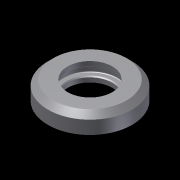
# Autodesk Inventor part: 機械油封墊片-KMB601PT-t10.4
Saved by Autodesk Inventor 2012 SP2 (Build 160219200, 219)
## iProperties
Created: 2015-05-11
Part Number: 機械油封墊片-KMB601PT-t10.4
Material: Default
Document SubType Name: Modeling
Designer: Eric
Density: 1 g/cm^3
Author: Eric
Autodesk Inventor part; units mm, degrees
ref_plane "YZ Plane" through (0, 0, 0) normal (1, 0, 0) x (0, 1, 0)
ref_plane "XZ Plane" through (0, 0, 0) normal (0, 1, 0) x (-1, 0, 0)
ref_plane "XY Plane" through (0, 0, 0) normal (0, 0, 1) x (1, 0, 0)
sketch "草圖1" plane through (0, 0, 0) normal (0, 0, 1) x (1, 0, 0)
  circle A0 centre (0, 0) radius 23.5
  dimension "d0" = 47
  constraints: 1 centre point, 1 coincident
  measures "d0" diameter of A0
extrude "擠出1" add sketch "草圖1" along normal blind 10.4
chamfer "倒角1" distance 3 angle 45 1 edges at (-23.5, 0, 10.4)
sketch "草圖3" plane through (0, 0, 10.4) normal (0, 0, 1) x (1, 0, 0)
  circle A0 centre (0, 0) radius 20.5 projected
hole "孔1" at (0, 0, 10.4) direction (0, 0, -1) diameter 25 end through all
sketch "草圖4" plane through (0, 0, 0) normal (0, 1, 0) x (-1, 0, 0)
  line L0 (0, 0) -> (0, 3)
  line L1 (-15.55, 7.4) -> (15.55, 7.4)
  line L2 (15.55, 7.4) -> (15.55, 3)
  line L3 (15.55, 3) -> (-15.55, 3)
  line L4 (-15.55, 3) -> (-15.55, 7.4)
  line L5 (0, 7.4) -> (0, 3)
  dimension "d13" = 3
  dimension "d14" = 31.1
  dimension "d15" = 4.4
  constraints: 12 end point, 2 midpoint, 2 parallel, 1 horizontal, 1 perpendicular, 1 vertical
  measures "d13" distance of L0.start L0.end
  measures "d14" distance of L2.end L3.end
  measures "d15" distance of L1.end L2.end
revolve "迴轉1" cut sketch "草圖4" angle 360 about axis through (0, 0, 7.4) along (0, 0, -1) contours L1 L2 L3 L5
fillet "圓角1" radius 0.5 2 edges at (15.55, 0, 3) (15.55, 0, 7.4)
chamfer "倒角2" distance 0.5 angle 45 2 edges at (0, 12.5, 7.4) (0, 12.5, 3)
